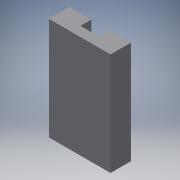
# Autodesk Inventor part: commutator_attachement_front_plate
Saved by Autodesk Inventor 2016 (Build 200138000, 138)
## iProperties
Created: 2016-09-28
Part Number: commutator_attachement_front_plate
Material: Generic
Document SubType Name: Modeling
Designer: ajar021
Density: 1 g/cm^3
Appearance: Default
Author: ajar021
Autodesk Inventor part; units mm, degrees
ref_plane "YZ Plane" through (0, 0, 0) normal (1, 0, 0) x (0, 1, 0)
ref_plane "XZ Plane" through (0, 0, 0) normal (0, 1, 0) x (-1, 0, 0)
ref_plane "XY Plane" through (0, 0, 0) normal (0, 0, 1) x (1, 0, 0)
sketch "Sketch1" plane through (0, 0, 0) normal (0, 0, 1) x (1, 0, 0)
  line L0 (-6, 10) -> (6, 10)
  line L1 (6, 10) -> (6, -10)
  line L2 (6, -10) -> (-6, -10)
  line L3 (-6, -10) -> (-6, 10)
  line L4 (-6, 10) -> (6, -10) construction
  line L5 (6, 10) -> (-6, -10) construction
  line L6 (0, 10) -> (0, -10) construction
  point P0 (0, 0)
  dimension "d0" = 12
  dimension "d1" = 20
  constraints: 14 end point, 4 midpoint, 2 parallel, 1 horizontal, 1 perpendicular
  measures "d0" distance of L0.start L0.end
  measures "d1" distance of L0.end L1.end
extrude "Extrusion1" add sketch "Sketch1" along normal blind 4
sketch "Sketch2" plane through (0, 0, 0) normal (0, 0, -1) x (-1, 0, 0)
  line L0 (-6, 10) -> (6, 10) projected
  line L1 (0, 10) -> (-1.75, 10)
  line L2 (-1.75, 10) -> (-1.75, 6.5)
  line L3 (-1.75, 6.5) -> (1.75, 6.5)
  line L4 (1.75, 6.5) -> (1.75, 10)
  line L5 (0, 10) -> (1.75, 10)
  line L6 (6, -10) -> (-6, -10) projected
  line L7 (-1.75, -10) -> (-1.75, -6.5)
  line L8 (-1.75, -6.5) -> (1.75, -6.5)
  line L9 (1.75, -6.5) -> (1.75, -10)
  line L10 (-1.75, -10) -> (1.75, -10)
  point P0 (0, 0)
  dimension "d5" = 1.75
  dimension "d6" = 1.75
  dimension "d7" = 3.5
  dimension "d8" = 3.5
  constraints: 18 end point, 6 perpendicular, 4 point on line, 2 collinear, 1 midpoint
  measures "d5" distance of L1.start L1.end
  measures "d6" distance of L4.end L1.start
  measures "d7" distance of L3.end L4.end
  measures "d8" distance of L7.start L7.end
extrude "Extrusion2" cut sketch "Sketch2" against normal blind 2.1
equation "\"d6\" = d5"
equation "\"d7\" = 2 * d5"
equation "\"d8\" = d7"
body "Solid1"
